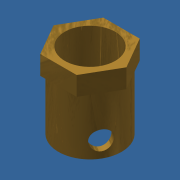
# Autodesk Inventor part: messingnut
Saved by Autodesk Inventor 2014 SP2 (Build 180246200, 246)
## iProperties
Created: 2015-01-19
Part Number: messingnut
Material: Messing, weicher Gelbton
Document SubType Name: Modeling
Designer: 4ndreas
Density: 8.47 g/cm^3
Appearance: Messing - satiniert
Author: 4ndreas
Autodesk Inventor part; units mm, degrees
ref_plane "YZ Plane" through (0, 0, 0) normal (1, 0, 0) x (0, 1, 0)
ref_plane "XZ Plane" through (0, 0, 0) normal (0, 1, 0) x (-1, 0, 0)
ref_plane "XY Plane" through (0, 0, 0) normal (0, 0, 1) x (1, 0, 0)
sketch "Skizze1" plane through (0, 0, 0) normal (0, 0, 1) x (1, 0, 0)
  circle A0 centre (0, 0) radius 5
  circle A1 centre (0, 0) radius 4
  dimension "d0" = 8
  dimension "d1" = 10
  constraints: 2 centre point, 2 coincident
  measures "d0" diameter of A1
  measures "d1" diameter of A0
extrude "Extrusion1" add sketch "Skizze1" along normal blind 12
sketch "Skizze2" plane through (0, 0, 12) normal (0, 0, 1) x (1, 0, 0)
  circle A0 centre (0, 0) radius 5 projected
  line L0 (-2.8868, 5) -> (2.8868, 5)
  line L1 (2.8868, 5) -> (5.7735, 0)
  line L2 (5.7735, 0) -> (2.8868, -5)
  line L3 (2.8868, -5) -> (-2.8868, -5)
  line L4 (-2.8868, -5) -> (-5.7735, 0)
  line L5 (-5.7735, 0) -> (-2.8868, 5)
  constraints: 12 end point, 1 coincident, 1 horizontal, 1 tangent, 13 other
extrude "Extrusion2" add sketch "Skizze2" against normal blind 3 contours A0 L1 L2 | A0 L0 L1 | L2 L3 A0 | A0 L5 L0 | L3 L4 A0 | A0 L4 L5
sketch "Skizze3" plane through (5.7735, 0, 12) normal (0.8660254, -0.5, 0) x (0, 0, -1)
  line L0 (0, 0) -> (0, -5.7735) projected
  line L1 (0, -2.8868) -> (12, -2.8868) construction
  point P0 (9.5, -2.8868)
  dimension "d6" = 2.5
  constraints: 2 end point, 1 midpoint, 1 point on line
  measures "d6" distance of point (9.5, -2.887) L1.end
hole "Bohrung1" at (4.3301, -2.5, 2.5) direction (-0.8660254, 0.5, 0) diameter 3 depth 4 tip angle 118
